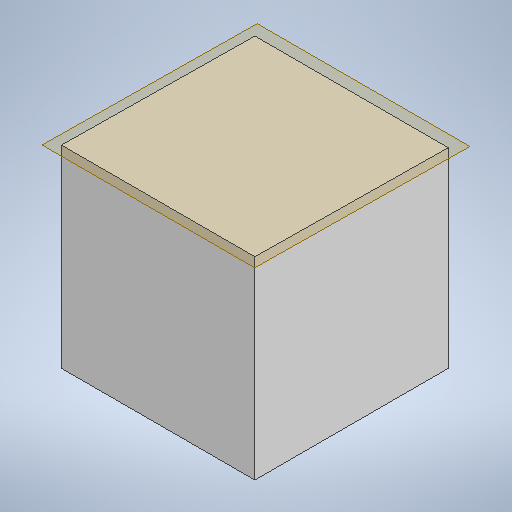
# Autodesk Inventor part: filler_cube
Saved by Autodesk Inventor 2025 (Build 290162000, 162)
## iProperties
Created: 2026-06-11
Part Number: filler_cube
Material: Generic
Document SubType Name: Modeling
Designer: DSTJOHN
Density: 1 g/cm^3
Appearance: Default
Author: DSTJOHN
Autodesk Inventor part; units mm, degrees
ref_plane "YZ Plane" through (0, 0, 0) normal (1, 0, 0) x (0, 1, 0)
ref_plane "XZ Plane" through (0, 0, 0) normal (0, 1, 0) x (-1, 0, 0)
ref_plane "XY Plane" through (0, 0, 0) normal (0, 0, 1) x (1, 0, 0)
sketch "Sketch1" plane through (0, 0, 0) normal (0, 1, 0) x (-1, 0, 0)
  line L0 (-25, 0) -> (-29, 0)
  line L1 (-29, 0) -> (-29, -4)
  line L2 (-29, -4) -> (-25, -4)
  line L3 (-25, -4) -> (-25, 0)
  line L4 (0, 0) -> (0, -8.4047) construction
  point P0 (-25, -2)
  dimension "d0" = 4
  dimension "d1" = 4
  dimension "d2" = 25
  constraints: 10 end point, 2 parallel, 1 horizontal, 1 midpoint, 1 perpendicular, 1 vertical
  measures "d0" distance of L2.end L1.end
  measures "d1" distance of L1.end L0.end
  measures "d2" distance from line of point (-25, -2) L4
extrude "Extrusion1" add sketch "Sketch1" along normal blind 4
ref_plane "Work Plane1" through (25, 4, 0) normal (0, 0.9999302, -0.0118156) x (1, 0, 0)
sketch "Sketch2" plane through (25, 4, 0) normal (0, 0.9999302, -0.0118156) x (1, 0, 0)
  line L0 (-0.8908, -1.2177) -> (5.211, -1.2177)
  line L1 (5.211, -1.2177) -> (5.211, 5.5983)
  line L2 (5.211, 5.5983) -> (-0.8908, 5.5983)
  line L3 (-0.8908, 5.5983) -> (-0.8908, -1.2177)
  point P0 (-25, 0.0473)
  constraints: 8 end point, 2 parallel, 1 horizontal, 1 perpendicular
extrude "Extrusion2" cut sketch "Sketch2" along normal blind 1.5
body "Solid1"
